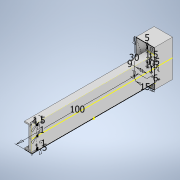
# Autodesk Inventor part: 3D_print_actuator_cable_driven
Saved by Autodesk Inventor 2021 (Build 250183000, 183)
## iProperties
Created: 2021-04-12
Part Number: 3D_print_actuator_cable_driven
Material: Generic
Document SubType Name: Modeling
Designer: Charlie
Density: 1 g/cm^3
Appearance: Default
Author: Charlie
Autodesk Inventor part; units mm, degrees
ref_plane "YZ Plane" through (0, 0, 0) normal (1, 0, 0) x (0, 1, 0)
ref_plane "XY Plane" through (0, 0, 0) normal (0, 0, 1) x (1, 0, 0)
sketch "Sketch1" plane through (0, 0, 0) normal (0, 1, 0) x (-1, 0, 0)
  line L0 (-3, 50) -> (3, 50)
  line L1 (3, 50) -> (3, -50)
  line L2 (3, -50) -> (-3, -50)
  line L3 (-3, -50) -> (-3, 50)
  line L4 (-3, 50) -> (3, -50) construction
  line L5 (3, 50) -> (-3, -50) construction
  point P0 (0, 0)
  dimension "d123" = 6
  dimension "d124" = 100
  constraints: 12 end point, 2 midpoint, 2 parallel, 1 horizontal, 1 perpendicular
  measures "d123" distance of L1.end L2.end
  measures "d124" distance of L0.end L1.end
extrude "Extrusion1" add sketch "Sketch1" along normal blind 20
sketch "Sketch2" plane through (0, 0, -50) normal (0, 0, -1) x (-1, 0, 0)
  line L0 (-3, 25) -> (12, 25)
  line L1 (12, 25) -> (12, -5)
  line L2 (12, -5) -> (-3, -5)
  line L3 (-3, -5) -> (-3, 25)
  line L4 (3, 0) -> (3, 20) projected
  line L5 (-3, 25) -> (12, -5) construction
  line L6 (12, 25) -> (-3, -5) construction
  line L7 (-3, 0) -> (-3, 20) projected
  line L8 (-3, 20) -> (3, 20) projected
  line L9 (0, 20) -> (0, 0) construction
  circle A0 centre (-1.5, 18.5) radius 0.5
  circle A1 centre (-1.5, 10) radius 0.5
  line L10 (-3, 10) -> (3, 10) construction
  circle A2 centre (-1.5, 1.5) radius 0.5
  line L11 (-0.5, 1) -> (-0.5, 19)
  dimension "d125" = 15
  dimension "d126" = 30
  dimension "d127" = 5
  dimension "d128" = 9
  dimension "d129" = 1
  dimension "d130" = 1.5
  dimension "d131" = 1.5
  dimension "d132" = 1
  dimension "d133" = 1.5
  dimension "d134" = 10
  constraints: 18 end point, 3 centre point, 3 midpoint, 2 horizontal, 2 parallel, 1 perpendicular, 1 symmetric about line, 1 vertical, 1 other
  measures "d125" distance of L1.end L2.end
  measures "d126" distance of L0.end L1.end
  measures "d127" distance between parallel lines of L0 L8
  measures "d128" distance between parallel lines of L4 L1
  measures "d129" diameter of A0
  measures "d130" distance from line of L3 A0.centre
  measures "d131" distance from line of A0.centre L8
  measures "d132" diameter of A1
  measures "d133" distance from line of L3 A1.centre
  measures "d134" distance from line of L8 A1.centre
extrude "Extrusion21" add sketch "Sketch2" along normal blind 15 contours L0 L1 L2 L3 | A0 | A1 | A2
extrude "Extrusion22" cut sketch "Sketch2" along normal blind 15 and the other way blind 100 contours A0 | A1 | A2
sketch "Sketch15" plane through (-3, 0, 50) normal (0, 0, 1) x (1, 0, 0)
  line L0 (3.5, 1) -> (-3.5, 1)
  line L1 (-3.5, 1) -> (-3.5, 19)
  line L2 (-3.5, 19) -> (3.5, 19)
  line L3 (3.5, 19) -> (3.5, 1)
  line L4 (0, 0) -> (0, 20) projected
  line L5 (3.5, 1) -> (-3.5, 19) construction
  line L6 (-3.5, 1) -> (3.5, 19) construction
  point P0 (3, 0)
  point P1 (0, 10)
  dimension "d145" = 7
  dimension "d146" = 18
  constraints: 12 end point, 3 midpoint, 2 parallel, 1 horizontal, 1 perpendicular
  measures "d145" distance of L1.end L2.end
  measures "d146" distance of L0.end L1.end
extrude "Extrusion24" cut sketch "Sketch15" against normal blind 100
sketch "Sketch16" plane through (3, 0, 50) normal (1, 0, 0) x (0, 0, -1)
  line L0 (100, 20) -> (0, 20) construction
  line L1 (4, 20) -> (4, 0) construction
  line L2 (100, 0) -> (0, 0) construction
  line L3 (0, 0) -> (0, 20) construction
  circle A0 centre (4, 18.5) radius 0.5
  line L4 (0, 10.5) -> (115, 10.5) projected
  circle A1 centre (4, 10.5) radius 0.5
  circle A2 centre (4, 1.5) radius 0.5
  point P0 (50, 0)
  dimension "d149" = 4
  dimension "d150" = 1
  dimension "d151" = 1
  dimension "d152" = 1.5
  dimension "d154" = 1
  dimension "d155" = 1.5
  constraints: 6 point on line, 3 centre point, 2 end point, 1 vertical
  measures "d149" distance between parallel lines of L1 L3
  measures "d150" diameter of A0
  measures "d151" diameter of A1
  measures "d152" distance from line of L0 A0.centre
  measures "d154" diameter of A2
  measures "d155" distance from line of L2 A2.centre
sketch "Sketch6" plane through (0, 10, 0) normal (0, 1, 0) x (-1, 0, 0)
  line L0 (21.0864, 109.726) -> (-9.863, 109.726)
  line L1 (-9.863, 109.726) -> (-9.863, -3.5286)
  line L2 (-9.863, -3.5286) -> (21.0864, -3.5286)
  line L3 (21.0864, -3.5286) -> (21.0864, 109.726)
  point P0 (0, 0)
  dimension "d36" = 113.2546
  dimension "d37" = 30.9494
  constraints: 8 end point, 2 parallel, 1 horizontal, 1 perpendicular
  measures "d36" distance of L2.end L0.start
  measures "d37" distance of L1.end L2.end
body "Solid1"
